Autodesk Inventor part; units mm, degrees
(part 3 of 4)
sketch "Sketch14" plane through (0, 0, 0) normal (0, 0, -1) x (-1, 0, 0)
  line L0 (-1.9956, 5.4384) -> (3.1347, 5.4384) construction
  line L1 (3.1347, 5.4384) -> (3.1347, -17.7526) construction
  line L2 (3.1347, -17.7526) -> (-1.9956, -17.7526) construction
  line L3 (-1.9956, -17.7526) -> (-1.9956, 5.4384) construction
  line L4 (4.75, -5.9162) -> (4.75, -5.8379)
  line L5 (4.75, -4.9221) -> (4.75, -4.8438)
  line L6 (5.6579, -4.9221) -> (5.6579, -5.8379)
  line L7 (4.75, -4.9221) -> (5.6579, -4.9221)
  line L8 (5.7362, -4.8438) -> (4.75, -4.8438)
  line L9 (5.7362, -5.9162) -> (5.7362, -4.8438)
  line L10 (5.6579, -5.8379) -> (4.75, -5.8379)
  line L11 (4.75, -5.9162) -> (5.7362, -5.9162)
  line L12 (4.55, -5.9162) -> (4.55, -5.8379)
  line L13 (4.55, -4.9221) -> (4.55, -4.8438)
  line L14 (4.55, -5.8379) -> (3.6421, -5.8379)
  line L15 (3.5638, -5.9162) -> (4.55, -5.9162)
  line L16 (3.6421, -4.9221) -> (4.55, -4.9221)
  line L17 (4.55, -4.8438) -> (3.5638, -4.8438)
  line L18 (3.6421, -5.8379) -> (3.6421, -4.9221)
  line L19 (3.5638, -4.8438) -> (3.5638, -5.9162)
  line L20 (4.55, -5.8379) -> (3.6421, -5.8379)
  line L21 (3.6421, -5.8379) -> (3.6421, -4.9221)
  line L22 (3.6421, -4.9221) -> (4.55, -4.9221)
  line L23 (4.55, -4.9221) -> (4.55, -4.8438)
  line L24 (4.55, -4.8438) -> (3.5638, -4.8438)
  line L25 (3.5638, -4.8438) -> (3.5638, -5.9162)
  line L26 (3.5638, -5.9162) -> (4.55, -5.9162)
  line L27 (4.55, -5.9162) -> (4.55, -5.8379)
  line L28 (4.75, -4.8438) -> (4.75, -4.9221)
  line L29 (4.75, -4.9221) -> (5.6579, -4.9221)
  line L30 (5.6579, -4.9221) -> (5.6579, -5.8379)
  line L31 (5.6579, -5.8379) -> (4.75, -5.8379)
  line L32 (4.75, -5.8379) -> (4.75, -5.9162)
  line L33 (4.75, -5.9162) -> (5.7362, -5.9162)
  line L34 (5.7362, -5.9162) -> (5.7362, -4.8438)
  line L35 (5.7362, -4.8438) -> (4.75, -4.8438)
  line L36 (-3.3239, 5.3849) -> (-3.3239, 5.4632)
  line L37 (-4.2318, 5.3849) -> (-3.3239, 5.3849)
  line L38 (-3.3239, 5.4632) -> (-4.3101, 5.4632)
  line L39 (-3.1239, 5.3849) -> (-3.1239, 5.4632)
  line L40 (-4.2318, 4.4692) -> (-4.2318, 5.3849)
  line L41 (-3.3239, 4.4692) -> (-4.2318, 4.4692)
  line L42 (-4.3101, 5.4632) -> (-4.3101, 4.3909)
  line L43 (-4.3101, 4.3909) -> (-3.3239, 4.3909)
  line L44 (-3.3239, 4.3909) -> (-3.3239, 4.4692)
  line L45 (-3.1239, 5.3849) -> (-2.2161, 5.3849)
  line L46 (-2.1378, 5.4632) -> (-3.1239, 5.4632)
  line L47 (-3.1239, 4.3909) -> (-3.1239, 4.4692)
  line L48 (-2.2161, 5.3849) -> (-2.2161, 4.4692)
  line L49 (-2.1378, 4.3909) -> (-2.1378, 5.4632)
  line L50 (-3.1239, 4.3909) -> (-2.1378, 4.3909)
  line L51 (-2.2161, 4.4692) -> (-3.1239, 4.4692)
  line L52 (-4.2318, 2.9331) -> (-4.2318, 3.8488)
  line L53 (-4.3101, 3.9271) -> (-4.3101, 2.8547)
  line L54 (-3.3239, 3.9271) -> (-4.3101, 3.9271)
  line L55 (-3.3239, 3.8488) -> (-3.3239, 3.9271)
  line L56 (-4.2318, 3.8488) -> (-3.3239, 3.8488)
  line L57 (-4.3101, 2.8547) -> (-3.3239, 2.8547)
  line L58 (-3.3239, 2.9331) -> (-4.2318, 2.9331)
  line L59 (-3.3239, 2.8547) -> (-3.3239, 2.9331)
  line L60 (-3.1239, 3.8488) -> (-3.1239, 3.9271)
  line L61 (-3.1239, 3.8488) -> (-2.2161, 3.8488)
  line L62 (-2.1378, 3.9271) -> (-3.1239, 3.9271)
  line L63 (-3.1239, 2.8547) -> (-3.1239, 2.9331)
  line L64 (-2.2161, 3.8488) -> (-2.2161, 2.9331)
  line L65 (-2.1378, 2.8547) -> (-2.1378, 3.9271)
  line L66 (-3.1239, 2.8547) -> (-2.1378, 2.8547)
  line L67 (-2.2161, 2.9331) -> (-3.1239, 2.9331)
  line L68 (-4.2318, 1.4571) -> (-4.2318, 2.3729)
  line L69 (-4.3101, 2.4512) -> (-4.3101, 1.3788)
  line L70 (-3.3239, 2.4512) -> (-4.3101, 2.4512)
  line L71 (-3.3239, 2.3729) -> (-3.3239, 2.4512)
  line L72 (-4.2318, 2.3729) -> (-3.3239, 2.3729)
  line L73 (-4.3101, 1.3788) -> (-3.3239, 1.3788)
  line L74 (-3.3239, 1.4571) -> (-4.2318, 1.4571)
  line L75 (-3.3239, 1.3788) -> (-3.3239, 1.4571)
  line L76 (-3.1239, 2.3729) -> (-3.1239, 2.4512)
  line L77 (-3.1239, 2.3729) -> (-2.2161, 2.3729)
  line L78 (-2.1378, 2.4512) -> (-3.1239, 2.4512)
  line L79 (-3.1239, 1.3788) -> (-3.1239, 1.4571)
  line L80 (-2.2161, 2.3729) -> (-2.2161, 1.4571)
  line L81 (-2.1378, 1.3788) -> (-2.1378, 2.4512)
  line L82 (-3.1239, 1.3788) -> (-2.1378, 1.3788)
  line L83 (-2.2161, 1.4571) -> (-3.1239, 1.4571)
  line L84 (-4.2318, -0.0188) -> (-4.2318, 0.8969)
  line L85 (-4.3101, 0.9753) -> (-4.3101, -0.0971)
  line L86 (-3.3239, 0.9753) -> (-4.3101, 0.9753)
  line L87 (-3.3239, 0.8969) -> (-3.3239, 0.9753)
  line L88 (-4.2318, 0.8969) -> (-3.3239, 0.8969)
  line L89 (-4.3101, -0.0971) -> (-3.3239, -0.0971)
  line L90 (-3.3239, -0.0188) -> (-4.2318, -0.0188)
  line L91 (-3.3239, -0.0971) -> (-3.3239, -0.0188)
  line L92 (-3.1239, 0.8969) -> (-3.1239, 0.9753)
  line L93 (-3.1239, 0.8969) -> (-2.2161, 0.8969)
  line L94 (-2.1378, 0.9753) -> (-3.1239, 0.9753)
  line L95 (-3.1239, -0.0971) -> (-3.1239, -0.0188)
  line L96 (-2.2161, 0.8969) -> (-2.2161, -0.0188)
  line L97 (-2.1378, -0.0971) -> (-2.1378, 0.9753)
  line L98 (-3.1239, -0.0971) -> (-2.1378, -0.0971)
  line L99 (-2.2161, -0.0188) -> (-3.1239, -0.0188)
  line L100 (-4.2318, -1.5262) -> (-4.2318, -0.6105)
  line L101 (-4.3101, -0.5322) -> (-4.3101, -1.6045)
  line L102 (-3.3239, -0.5322) -> (-4.3101, -0.5322)
  line L103 (-3.3239, -0.6105) -> (-3.3239, -0.5322)
  line L104 (-4.2318, -0.6105) -> (-3.3239, -0.6105)
  line L105 (-4.3101, -1.6045) -> (-3.3239, -1.6045)
  line L106 (-3.3239, -1.5262) -> (-4.2318, -1.5262)
  line L107 (-3.3239, -1.6045) -> (-3.3239, -1.5262)
  line L108 (-3.1239, -0.6105) -> (-3.1239, -0.5322)
  line L109 (-3.1239, -0.6105) -> (-2.2161, -0.6105)
  line L110 (-2.1378, -0.5322) -> (-3.1239, -0.5322)
  line L111 (-3.1239, -1.6045) -> (-3.1239, -1.5262)
  line L112 (-2.2161, -0.6105) -> (-2.2161, -1.5262)
  line L113 (-2.1378, -1.6045) -> (-2.1378, -0.5322)
  line L114 (-3.1239, -1.6045) -> (-2.1378, -1.6045)
  line L115 (-2.2161, -1.5262) -> (-3.1239, -1.5262)
  spline S0 degree 2 poles (-1.4607, 4.3962) (-1.686, 4.3962) (-1.9502, 4.6685) (-1.9502, 4.9149) knots 0 0 0 1 2 2 2
  spline S1 degree 2 poles (-1.9502, 4.9149) (-1.9502, 5.1523) (-1.6852, 5.4351) (-1.4599, 5.4351) knots 0 0 0 1 2 2 2
  spline S2 degree 2 poles (-1.4599, 5.4351) (-1.4007, 5.4351) (-1.3051, 5.4214) (-1.2614, 5.41) knots 0 0 0 1 2 2 2
  spline S3 degree 2 poles (-1.2614, 5.41) (-1.2273, 5.3995) (-1.1471, 5.3646) (-1.122, 5.3517) knots 0 0 0 1 2 2 2
  line L116 (-1.122, 5.3517) -> (-1.122, 5.1134)
  line L117 (-1.122, 5.1134) -> (-1.1471, 5.1134)
  spline S4 degree 2 poles (-1.1471, 5.1134) (-1.1657, 5.1296) (-1.2208, 5.175) (-1.2557, 5.1961) knots 0 0 0 1 2 2 2
  spline S5 degree 2 poles (-1.2557, 5.1961) (-1.2905, 5.218) (-1.374, 5.2479) (-1.4202, 5.2479) knots 0 0 0 1 2 2 2
  spline S6 degree 2 poles (-1.4202, 5.2479) (-1.4745, 5.2479) (-1.5644, 5.2139) (-1.6058, 5.171) knots 0 0 0 1 2 2 2
  spline S7 degree 2 poles (-1.6058, 5.171) (-1.643, 5.1329) (-1.6909, 5.0024) (-1.6909, 4.9141) knots 0 0 0 1 2 2 2
  spline S8 degree 2 poles (-1.6909, 4.9141) (-1.6909, 4.8209) (-1.6414, 4.6936) (-1.6009, 4.6547) knots 0 0 0 1 2 2 2
  spline S9 degree 2 poles (-1.6009, 4.6547) (-1.562, 4.6167) (-1.4664, 4.5834) (-1.4186, 4.5834) knots 0 0 0 1 2 2 2
  spline S10 degree 2 poles (-1.4186, 4.5834) (-1.3691, 4.5834) (-1.2792, 4.6167) (-1.2484, 4.6369) knots 0 0 0 1 2 2 2
  spline S11 degree 2 poles (-1.2484, 4.6369) (-1.2144, 4.6572) (-1.1633, 4.7001) (-1.1447, 4.7171) knots 0 0 0 1 2 2 2
  line L118 (-1.1447, 4.7171) -> (-1.122, 4.7171)
  line L119 (-1.122, 4.7171) -> (-1.122, 4.4821)
  spline S12 degree 2 poles (-1.122, 4.4821) (-1.1495, 4.4692) (-1.2216, 4.4368) (-1.2605, 4.4254) knots 0 0 0 1 2 2 2
  spline S13 degree 2 poles (-1.2605, 4.4254) (-1.3075, 4.4108) (-1.3894, 4.3962) (-1.4607, 4.3962) knots 0 0 0 1 2 2 2
  spline S14 degree 2 poles (-0.2435, 4.6936) (-0.2435, 4.6296) (-0.297, 4.5186) (-0.3481, 4.4781) knots 0 0 0 1 2 2 2
  spline S15 degree 2 poles (-0.3481, 4.4781) (-0.3991, 4.4376) (-0.5458, 4.3922) (-0.6406, 4.3922) knots 0 0 0 1 2 2 2
  spline S16 degree 2 poles (-0.6406, 4.3922) (-0.7419, 4.3922) (-0.8934, 4.4384) (-0.9421, 4.4781) knots 0 0 0 1 2 2 2
  spline S17 degree 2 poles (-0.9421, 4.4781) (-0.9899, 4.5178) (-1.0353, 4.6256) (-1.0353, 4.6855) knots 0 0 0 1 2 2 2
  spline S18 degree 2 poles (-1.0353, 4.6855) (-1.0353, 4.7714) (-0.9404, 4.8857) (-0.8505, 4.9238) knots 0 0 0 1 2 2 2
  line L120 (-0.8505, 4.9238) -> (-0.8505, 4.9278)
  spline S19 degree 2 poles (-0.8505, 4.9278) (-0.9388, 4.9708) (-1.0085, 5.0932) (-1.0085, 5.1685) knots 0 0 0 1 2 2 2
  spline S20 degree 2 poles (-1.0085, 5.1685) (-1.0085, 5.2236) (-0.9599, 5.3201) (-0.9121, 5.3581) knots 0 0 0 1 2 2 2
  spline S21 degree 2 poles (-0.9121, 5.3581) (-0.8659, 5.3946) (-0.7257, 5.4384) (-0.6382, 5.4384) knots 0 0 0 1 2 2 2
  spline S22 degree 2 poles (-0.6382, 5.4384) (-0.5458, 5.4384) (-0.408, 5.3987) (-0.3635, 5.3663) knots 0 0 0 1 2 2 2
  spline S23 degree 2 poles (-0.3635, 5.3663) (-0.3181, 5.3338) (-0.2695, 5.2398) (-0.2695, 5.1855) knots 0 0 0 1 2 2 2
  spline S24 degree 2 poles (-0.2695, 5.1855) (-0.2695, 5.1142) (-0.3521, 5) (-0.4372, 4.9603) knots 0 0 0 1 2 2 2
  line L121 (-0.4372, 4.9603) -> (-0.4372, 4.957)
  spline S25 degree 2 poles (-0.4372, 4.957) (-0.3375, 4.9165) (-0.2435, 4.7852) (-0.2435, 4.6936) knots 0 0 0 1 2 2 2
  spline S26 degree 2 poles (-0.4915, 4.6831) (-0.4915, 4.7325) (-0.5336, 4.7844) (-0.6017, 4.8176) knots 0 0 0 1 2 2 2
  spline S27 degree 2 poles (-0.6017, 4.8176) (-0.6212, 4.8265) (-0.6949, 4.8549) (-0.7233, 4.8671) knots 0 0 0 1 2 2 2
  spline S28 degree 2 poles (-0.7233, 4.8671) (-0.7492, 4.8411) (-0.7905, 4.7633) (-0.7905, 4.7171) knots 0 0 0 1 2 2 2
  spline S29 degree 2 poles (-0.7905, 4.7171) (-0.7905, 4.6475) (-0.7014, 4.564) (-0.6293, 4.564) knots 0 0 0 1 2 2 2
  spline S30 degree 2 poles (-0.6293, 4.564) (-0.609, 4.564) (-0.5588, 4.5769) (-0.5393, 4.5899) knots 0 0 0 1 2 2 2
  spline S31 degree 2 poles (-0.5393, 4.5899) (-0.5174, 4.6053) (-0.4915, 4.6475) (-0.4915, 4.6831) knots 0 0 0 1 2 2 2
  spline S32 degree 2 poles (-0.5134, 5.1564) (-0.5134, 5.2074) (-0.5806, 5.2682) (-0.6382, 5.2682) knots 0 0 0 1 2 2 2
  spline S33 degree 2 poles (-0.6382, 5.2682) (-0.6933, 5.2682) (-0.7605, 5.2131) (-0.7605, 5.1726) knots 0 0 0 1 2 2 2
  spline S34 degree 2 poles (-0.7605, 5.1726) (-0.7605, 5.1329) (-0.72, 5.0834) (-0.6771, 5.0632) knots 0 0 0 1 2 2 2
  spline S35 degree 2 poles (-0.6771, 5.0632) (-0.6584, 5.0534) (-0.6066, 5.0332) (-0.5636, 5.017) knots 0 0 0 1 2 2 2
  spline S36 degree 2 poles (-0.5636, 5.017) (-0.5377, 5.051) (-0.5134, 5.115) (-0.5134, 5.1564) knots 0 0 0 1 2 2 2
  spline S37 degree 2 poles (-0.9996, 3.4149) (-0.9996, 3.2747) (-1.122, 3.0543) (-1.2152, 2.9951) knots 0 0 0 1 2 2 2
  spline S38 degree 2 poles (-1.2152, 2.9951) (-1.293, 2.9449) (-1.4761, 2.9157) (-1.579, 2.9157) knots 0 0 0 1 2 2 2
  line L122 (-1.579, 2.9157) -> (-1.8918, 2.9157)
  line L123 (-1.8918, 2.9157) -> (-1.8918, 3.9157)
  line L124 (-1.8918, 3.9157) -> (-1.5823, 3.9157)
  spline S39 degree 2 poles (-1.5823, 3.9157) (-1.4769, 3.9157) (-1.293, 3.8889) (-1.2119, 3.8371) knots 0 0 0 1 2 2 2
  spline S40 degree 2 poles (-1.2119, 3.8371) (-1.1139, 3.7739) (-0.9996, 3.5599) (-0.9996, 3.4149) knots 0 0 0 1 2 2 2
  spline S41 degree 2 poles (-1.2573, 3.4165) (-1.2573, 3.5154) (-1.3254, 3.6564) (-1.3951, 3.6961) knots 0 0 0 1 2 2 2
  spline S42 degree 2 poles (-1.3951, 3.6961) (-1.4461, 3.7236) (-1.5579, 3.7293) (-1.6357, 3.7293) knots 0 0 0 1 2 2 2
  line L125 (-1.6357, 3.7293) -> (-1.6406, 3.7293)
  line L126 (-1.6406, 3.7293) -> (-1.6406, 3.1029)
  line L127 (-1.6406, 3.1029) -> (-1.6357, 3.1029)
  spline S43 degree 2 poles (-1.6357, 3.1029) (-1.5515, 3.1029) (-1.4356, 3.1086) (-1.3829, 3.1418) knots 0 0 0 1 2 2 2
  spline S44 degree 2 poles (-1.3829, 3.1418) (-1.3213, 3.1807) (-1.2573, 3.3176) (-1.2573, 3.4165) knots 0 0 0 1 2 2 2
  line L128 (-0.1625, 2.9157) -> (-0.8229, 2.9157)
  line L129 (-0.8229, 2.9157) -> (-0.8229, 3.0899)
  line L130 (-0.8229, 3.0899) -> (-0.6122, 3.0899)
  line L131 (-0.6122, 3.0899) -> (-0.6122, 3.6191)
  line L132 (-0.6122, 3.6191) -> (-0.8229, 3.6191)
  line L133 (-0.8229, 3.6191) -> (-0.8229, 3.782)
  spline S45 degree 2 poles (-0.8229, 3.782) (-0.7767, 3.782) (-0.6852, 3.7941) (-0.6576, 3.8071) knots 0 0 0 1 2 2 2
  spline S46 degree 2 poles (-0.6576, 3.8071) (-0.626, 3.8233) (-0.5904, 3.8776) (-0.5871, 3.9181) knots 0 0 0 1 2 2 2
  line L134 (-0.5871, 3.9181) -> (-0.3683, 3.9181)
  line L135 (-0.3683, 3.9181) -> (-0.3683, 3.0899)
  line L136 (-0.3683, 3.0899) -> (-0.1625, 3.0899)
  line L137 (-0.1625, 3.0899) -> (-0.1625, 2.9157)
  line L138 (-0.968, 1.4157) -> (-1.2735, 1.4157)
  line L139 (-1.2735, 1.4157) -> (-1.5515, 1.7828)
  line L140 (-1.5515, 1.7828) -> (-1.6422, 1.7828)
  line L141 (-1.6422, 1.7828) -> (-1.6422, 1.4157)
  line L142 (-1.6422, 1.4157) -> (-1.8918, 1.4157)
  line L143 (-1.8918, 1.4157) -> (-1.8918, 2.4157)
  line L144 (-1.8918, 2.4157) -> (-1.4899, 2.4157)
  spline S47 degree 2 poles (-1.4899, 2.4157) (-1.4064, 2.4157) (-1.2832, 2.3946) (-1.2306, 2.3622) knots 0 0 0 1 2 2 2
  spline S48 degree 2 poles (-1.2306, 2.3622) (-1.1771, 2.3282) (-1.1139, 2.222) (-1.1139, 2.141) knots 0 0 0 1 2 2 2
  spline S49 degree 2 poles (-1.1139, 2.141) (-1.1139, 2.0267) (-1.2176, 1.8833) (-1.3043, 1.8411) knots 0 0 0 1 2 2 2
  line L145 (-1.3043, 1.8411) -> (-0.968, 1.4157)
  spline S50 degree 2 poles (-1.3716, 2.1094) (-1.3716, 2.1475) (-1.4007, 2.2017) (-1.434, 2.2163) knots 0 0 0 1 2 2 2
  spline S51 degree 2 poles (-1.434, 2.2163) (-1.4575, 2.2261) (-1.515, 2.2317) (-1.5579, 2.2317) knots 0 0 0 1 2 2 2
  line L146 (-1.5579, 2.2317) -> (-1.6422, 2.2317)
  line L147 (-1.6422, 2.2317) -> (-1.6422, 1.9627)
  line L148 (-1.6422, 1.9627) -> (-1.5701, 1.9627)
  spline S52 degree 2 poles (-1.5701, 1.9627) (-1.5182, 1.9627) (-1.4445, 1.9757) (-1.4194, 1.9959) knots 0 0 0 1 2 2 2
  spline S53 degree 2 poles (-1.4194, 1.9959) (-1.3951, 2.0154) (-1.3716, 2.0672) (-1.3716, 2.1094) knots 0 0 0 1 2 2 2
  line L149 (-0.1609, 1.4157) -> (-0.8959, 1.4157)
  line L150 (-0.8959, 1.4157) -> (-0.8959, 1.5786)
  spline S54 degree 2 poles (-0.8959, 1.5786) (-0.8027, 1.6531) (-0.6536, 1.7844) (-0.5977, 1.8436) knots 0 0 0 1 2 2 2
  spline S55 degree 2 poles (-0.5977, 1.8436) (-0.5239, 1.9205) (-0.4583, 2.0381) (-0.4583, 2.0996) knots 0 0 0 1 2 2 2
  spline S56 degree 2 poles (-0.4583, 2.0996) (-0.4583, 2.1693) (-0.5417, 2.2439) (-0.6163, 2.2439) knots 0 0 0 1 2 2 2
  spline S57 degree 2 poles (-0.6163, 2.2439) (-0.6544, 2.2439) (-0.7225, 2.2252) (-0.7573, 2.2107) knots 0 0 0 1 2 2 2
  spline S58 degree 2 poles (-0.7573, 2.2107) (-0.7913, 2.1953) (-0.84, 2.1628) (-0.8521, 2.1547) knots 0 0 0 1 2 2 2
  line L151 (-0.8521, 2.1547) -> (-0.8716, 2.1547)
  line L152 (-0.8716, 2.1547) -> (-0.8716, 2.3727)
  spline S59 degree 2 poles (-0.8716, 2.3727) (-0.8294, 2.393) (-0.6495, 2.4351) (-0.5661, 2.4351) knots 0 0 0 1 2 2 2
  spline S60 degree 2 poles (-0.5661, 2.4351) (-0.3878, 2.4351) (-0.2046, 2.2763) (-0.2046, 2.1329) knots 0 0 0 1 2 2 2
  spline S61 degree 2 poles (-0.2046, 2.1329) (-0.2046, 2.0445) (-0.2881, 1.8744) (-0.3845, 1.7771) knots 0 0 0 1 2 2 2
  spline S62 degree 2 poles (-0.3845, 1.7771) (-0.4453, 1.7171) (-0.5596, 1.6239) (-0.5847, 1.6045) knots 0 0 0 1 2 2 2
  line L153 (-0.5847, 1.6045) -> (-0.1609, 1.6045)
  line L154 (-0.1609, 1.6045) -> (-0.1609, 1.4157)
  line L155 (-0.968, -0.0843) -> (-1.2735, -0.0843)
  line L156 (-1.2735, -0.0843) -> (-1.5515, 0.2828)
  line L157 (-1.5515, 0.2828) -> (-1.6422, 0.2828)
  line L158 (-1.6422, 0.2828) -> (-1.6422, -0.0843)
  line L159 (-1.6422, -0.0843) -> (-1.8918, -0.0843)
  line L160 (-1.8918, -0.0843) -> (-1.8918, 0.9157)
  line L161 (-1.8918, 0.9157) -> (-1.4899, 0.9157)
  spline S63 degree 2 poles (-1.4899, 0.9157) (-1.4064, 0.9157) (-1.2832, 0.8946) (-1.2306, 0.8622) knots 0 0 0 1 2 2 2
  spline S64 degree 2 poles (-1.2306, 0.8622) (-1.1771, 0.8282) (-1.1139, 0.722) (-1.1139, 0.641) knots 0 0 0 1 2 2 2
  spline S65 degree 2 poles (-1.1139, 0.641) (-1.1139, 0.5267) (-1.2176, 0.3833) (-1.3043, 0.3411) knots 0 0 0 1 2 2 2
  line L162 (-1.3043, 0.3411) -> (-0.968, -0.0843)
  spline S66 degree 2 poles (-1.3716, 0.6094) (-1.3716, 0.6475) (-1.4007, 0.7017) (-1.434, 0.7163) knots 0 0 0 1 2 2 2
  spline S67 degree 2 poles (-1.434, 0.7163) (-1.4575, 0.7261) (-1.515, 0.7317) (-1.5579, 0.7317) knots 0 0 0 1 2 2 2
  line L163 (-1.5579, 0.7317) -> (-1.6422, 0.7317)
  line L164 (-1.6422, 0.7317) -> (-1.6422, 0.4627)
  line L165 (-1.6422, 0.4627) -> (-1.5701, 0.4627)
  spline S68 degree 2 poles (-1.5701, 0.4627) (-1.5182, 0.4627) (-1.4445, 0.4757) (-1.4194, 0.4959) knots 0 0 0 1 2 2 2
  spline S69 degree 2 poles (-1.4194, 0.4959) (-1.3951, 0.5154) (-1.3716, 0.5672) (-1.3716, 0.6094) knots 0 0 0 1 2 2 2
  spline S70 degree 2 poles (-0.186, 0.2188) (-0.186, 0.145) (-0.2403, 0.0243) (-0.293, -0.0179) knots 0 0 0 1 2 2 2
  spline S71 degree 2 poles (-0.293, -0.0179) (-0.3456, -0.06) (-0.4891, -0.1054) (-0.592, -0.1054) knots 0 0 0 1 2 2 2
  spline S72 degree 2 poles (-0.592, -0.1054) (-0.7087, -0.1054) (-0.8756, -0.0665) (-0.9283, -0.0422) knots 0 0 0 1 2 2 2
  line L166 (-0.9283, -0.0422) -> (-0.9283, 0.175)
  line L167 (-0.9283, 0.175) -> (-0.904, 0.175)
  spline S73 degree 2 poles (-0.904, 0.175) (-0.8489, 0.1402) (-0.7006, 0.0883) (-0.639, 0.0883) knots 0 0 0 1 2 2 2
  spline S74 degree 2 poles (-0.639, 0.0883) (-0.6025, 0.0883) (-0.5174, 0.1013) (-0.4883, 0.1223) knots 0 0 0 1 2 2 2
  spline S75 degree 2 poles (-0.4883, 0.1223) (-0.4656, 0.1393) (-0.438, 0.1888) (-0.438, 0.2333) knots 0 0 0 1 2 2 2
  spline S76 degree 2 poles (-0.438, 0.2333) (-0.438, 0.2779) (-0.4769, 0.3257) (-0.5093, 0.3371) knots 0 0 0 1 2 2 2
  spline S77 degree 2 poles (-0.5093, 0.3371) (-0.5417, 0.3484) (-0.6317, 0.3509) (-0.6665, 0.3509) knots 0 0 0 1 2 2 2
  line L168 (-0.6665, 0.3509) -> (-0.7095, 0.3509)
  line L169 (-0.7095, 0.3509) -> (-0.7095, 0.5267)
  line L170 (-0.7095, 0.5267) -> (-0.6698, 0.5267)
  spline S78 degree 2 poles (-0.6698, 0.5267) (-0.6244, 0.5267) (-0.5474, 0.5348) (-0.5207, 0.547) knots 0 0 0 1 2 2 2
  spline S79 degree 2 poles (-0.5207, 0.547) (-0.4939, 0.5599) (-0.4639, 0.6053) (-0.4639, 0.6442) knots 0 0 0 1 2 2 2
  spline S80 degree 2 poles (-0.4639, 0.6442) (-0.4639, 0.675) (-0.4923, 0.7131) (-0.5126, 0.7236) knots 0 0 0 1 2 2 2
  spline S81 degree 2 poles (-0.5126, 0.7236) (-0.5369, 0.7358) (-0.6017, 0.7439) (-0.6244, 0.7439) knots 0 0 0 1 2 2 2
  spline S82 degree 2 poles (-0.6244, 0.7439) (-0.6609, 0.7439) (-0.7379, 0.7269) (-0.7735, 0.7131) knots 0 0 0 1 2 2 2
  spline S83 degree 2 poles (-0.7735, 0.7131) (-0.8019, 0.7026) (-0.8635, 0.6685) (-0.878, 0.6596) knots 0 0 0 1 2 2 2
  line L171 (-0.878, 0.6596) -> (-0.8991, 0.6596)
  line L172 (-0.8991, 0.6596) -> (-0.8991, 0.8735)
  spline S84 degree 2 poles (-0.8991, 0.8735) (-0.8473, 0.8954) (-0.6722, 0.9368) (-0.5806, 0.9368) knots 0 0 0 1 2 2 2
  spline S85 degree 2 poles (-0.5806, 0.9368) (-0.4915, 0.9368) (-0.3602, 0.906) (-0.314, 0.876) knots 0 0 0 1 2 2 2
  spline S86 degree 2 poles (-0.314, 0.876) (-0.263, 0.8444) (-0.2119, 0.7471) (-0.2119, 0.6863) knots 0 0 0 1 2 2 2
  spline S87 degree 2 poles (-0.2119, 0.6863) (-0.2119, 0.6004) (-0.3108, 0.4724) (-0.3918, 0.4538) knots 0 0 0 1 2 2 2
  line L173 (-0.3918, 0.4538) -> (-0.3918, 0.444)
  spline S88 degree 2 poles (-0.3918, 0.444) (-0.3562, 0.4392) (-0.2881, 0.4133) (-0.2557, 0.3841) knots 0 0 0 1 2 2 2
  spline S89 degree 2 poles (-0.2557, 0.3841) (-0.2257, 0.3581) (-0.186, 0.2755) (-0.186, 0.2188) knots 0 0 0 1 2 2 2
  line L174 (-0.968, -1.5843) -> (-1.2735, -1.5843)
  line L175 (-1.2735, -1.5843) -> (-1.5515, -1.2172)
  line L176 (-1.5515, -1.2172) -> (-1.6422, -1.2172)
  line L177 (-1.6422, -1.2172) -> (-1.6422, -1.5843)
  line L178 (-1.6422, -1.5843) -> (-1.8918, -1.5843)
  line L179 (-1.8918, -1.5843) -> (-1.8918, -0.5843)
  line L180 (-1.8918, -0.5843) -> (-1.4899, -0.5843)
  spline S90 degree 2 poles (-1.4899, -0.5843) (-1.4064, -0.5843) (-1.2832, -0.6054) (-1.2306, -0.6378) knots 0 0 0 1 2 2 2
  spline S91 degree 2 poles (-1.2306, -0.6378) (-1.1771, -0.6718) (-1.1139, -0.778) (-1.1139, -0.859) knots 0 0 0 1 2 2 2
  spline S92 degree 2 poles (-1.1139, -0.859) (-1.1139, -0.9733) (-1.2176, -1.1167) (-1.3043, -1.1589) knots 0 0 0 1 2 2 2
  line L181 (-1.3043, -1.1589) -> (-0.968, -1.5843)
  spline S93 degree 2 poles (-1.3716, -0.8906) (-1.3716, -0.8525) (-1.4007, -0.7983) (-1.434, -0.7837) knots 0 0 0 1 2 2 2
  spline S94 degree 2 poles (-1.434, -0.7837) (-1.4575, -0.7739) (-1.515, -0.7683) (-1.5579, -0.7683) knots 0 0 0 1 2 2 2
  line L182 (-1.5579, -0.7683) -> (-1.6422, -0.7683)
  line L183 (-1.6422, -0.7683) -> (-1.6422, -1.0373)
  line L184 (-1.6422, -1.0373) -> (-1.5701, -1.0373)
  spline S95 degree 2 poles (-1.5701, -1.0373) (-1.5182, -1.0373) (-1.4445, -1.0243) (-1.4194, -1.0041) knots 0 0 0 1 2 2 2
  spline S96 degree 2 poles (-1.4194, -1.0041) (-1.3951, -0.9846) (-1.3716, -0.9328) (-1.3716, -0.8906) knots 0 0 0 1 2 2 2
  line L185 (-0.1487, -1.3509) -> (-0.284, -1.3509)
  line L186 (-0.284, -1.3509) -> (-0.284, -1.5867)
  line L187 (-0.284, -1.5867) -> (-0.5263, -1.5867)
  line L188 (-0.5263, -1.5867) -> (-0.5263, -1.3509)
  line L189 (-0.5263, -1.3509) -> (-0.9672, -1.3509)
  line L190 (-0.9672, -1.3509) -> (-0.9672, -1.1645)
  line L191 (-0.9672, -1.1645) -> (-0.5344, -0.5843)
  line L192 (-0.5344, -0.5843) -> (-0.284, -0.5843)
  line L193 (-0.284, -0.5843) -> (-0.284, -1.171)
  line L194 (-0.284, -1.171) -> (-0.1487, -1.171)
  line L195 (-0.1487, -1.171) -> (-0.1487, -1.3509)
  line L196 (-0.5263, -1.171) -> (-0.5263, -0.8307)
  line L197 (-0.5263, -0.8307) -> (-0.78, -1.171)
  line L198 (-0.78, -1.171) -> (-0.5263, -1.171)
  point P0 (0, 0)
  point P1 (5.6, -4.98)
  point P2 (-2.2739, 5.3271)
  point P3 (-2.2739, 3.7909)
  point P4 (-2.2739, 2.315)
  point P5 (-2.2739, 0.8391)
  point P6 (-2.2739, -0.6684)
  constraints: 192 end point, 2 other
extrude "Extrusion14" add sketch "Sketch14" along normal blind 0.1 separate body contours L37 L40 L41 L44 L43 L42 L38 L36 | L39 L46 L49 L50 L47 L51 L48 L45 | L58 L59 L57 L53 L54 L55 L56 L52 | L60 L62 L65 L66 L63 L67 L64 L61 | L74 L75 L73 L69 L70 L71 L72 L68 | L76 L78 L81 L82 L79 L83 L80 L77 | L90 L91 L89 L85 L86 L87 L88 L84 | L92 L94 L97 L98 L95 L99 L96 L93 | L106 L107 L105 L101 L102 L103 L104 L100 | L108 L110 L113 L114 L111 L115 L112 L109 | S0 S1 S2 S3 L116 L117 S4 S5 S6 S7 S8 S9 S10 S11 L118 L119 S12 S13 | S14 S15 S16 S17 S18 L120 S19 S20 S21 S22 S23 S24 L121 S25 | S37 S38 L122 L123 L124 S39 S40 | L128 L129 L130 L131 L132 L133 S45 S46 L134 L135 L136 L137 | L138 L139 L140 L141 L142 L143 L144 S47 S48 S49 L145 | L149 L150 S54 S55 S56 S57 S58 L151 L152 S59 S60 S61 S62 L153 L154 | L155 L156 L157 L158 L159 L160 L161 S63 S64 S65 L162 | S70 S71 S72 L166 L167 S73 S74 S75 S76 S77 L168 L169 L170 S78 S79 S80 S81 S82 S83 L171 L172 S84 S85 S86 S87 L173 S88 S89 | L174 L175 L176 L177 L178 L179 L180 S90 S91 S92 L181 | L185 L186 L187 L188 L189 L190 L191 L192 L193 L194 L195
sketch "Sketch15" plane through (0, 0, 0) normal (0, 0, -1) x (-1, 0, 0)
  line L0 (3.7, 1.72) -> (3.7, 0.92)
  line L1 (5.6, 1.72) -> (3.7, 1.72)
  line L2 (3.7, 0.92) -> (5.6, 0.92)
  line L3 (5.6, 0.92) -> (5.6, 1.72)
  line L4 (-4.2318, 5.3849) -> (-3.3239, 5.3849)
  line L5 (-4.2318, 5.3849) -> (-2.2161, 5.3849)
  line L6 (-2.2161, 4.4692) -> (-3.1239, 4.4692)
  line L7 (-2.2161, 5.3849) -> (-2.2161, 4.4692)
  line L8 (-4.2318, 4.4692) -> (-4.2318, 5.3849)
  line L9 (-2.2161, 4.4692) -> (-4.2318, 4.4692)
  line L10 (-4.2318, 4.4692) -> (-4.2318, 5.3849)
  line L11 (-2.2907, 5.3103) -> (-4.1571, 5.3103)
  line L12 (-4.1571, 5.3103) -> (-4.1571, 4.5439)
  line L13 (-4.1571, 4.5439) -> (-2.2907, 4.5439)
  line L14 (-2.2907, 4.5439) -> (-2.2907, 5.3103)
  line L15 (-2.2907, 3.7924) -> (-4.1571, 3.7924)
  line L16 (-4.1571, 3.7924) -> (-4.1571, 3.026)
  line L17 (-4.1571, 3.026) -> (-2.2907, 3.026)
  line L18 (-2.2907, 3.026) -> (-2.2907, 3.7924)
  line L19 (-2.2907, 2.3165) -> (-4.1571, 2.3165)
  line L20 (-4.1571, 2.3165) -> (-4.1571, 1.5501)
  line L21 (-4.1571, 1.5501) -> (-2.2907, 1.5501)
  line L22 (-2.2907, 1.5501) -> (-2.2907, 2.3165)
  line L23 (-2.2907, 0.8182) -> (-4.1571, 0.8182)
  line L24 (-4.1571, 0.8182) -> (-4.1571, 0.0518)
  line L25 (-4.1571, 0.0518) -> (-2.2907, 0.0518)
  line L26 (-2.2907, 0.0518) -> (-2.2907, 0.8182)
  line L27 (-2.2907, -0.6669) -> (-4.1571, -0.6669)
  line L28 (-4.1571, -0.6669) -> (-4.1571, -1.4333)
  line L29 (-4.1571, -1.4333) -> (-2.2907, -1.4333)
  line L30 (-2.2907, -1.4333) -> (-2.2907, -0.6669)
  point P0 (0, 0)
  point P1 (-2.2161, 2.9331)
  point P2 (-2.2161, 1.4571)
  point P3 (-2.2161, -0.0188)
  point P4 (-2.2161, -1.5262)
  constraints: 48 end point, 18 perpendicular, 1 horizontal, 3 other
extrude "Extrusion15" add sketch "Sketch15" along normal up to surface (1 mm away) separate body contours L14 L13 L12 L11 | L18 L17 L16 L15 | L22 L21 L20 L19 | L26 L25 L24 L23 | L30 L29 L28 L27
chamfer "Chamfer4" distance 0.1 angle 45 20 edges at (4.1571, 1.9333, -1) (3.2239, 1.5501, -1) (2.2907, 1.9333, -1) (3.2239, 2.3165, -1) (4.1571, 0.435, -1) (3.2239, 0.0518, -1) (2.2907, 0.435, -1) (3.2239, 0.8182, -1) (4.1571, -1.0501, -1) (3.2239, -0.6669, -1) (3.2239, -1.4333, -1) (2.2907, -1.0501, -1) (4.1571, 3.4092, -1) (3.2239, 3.026, -1) (2.2907, 3.4092, -1) (3.2239, 3.7924, -1) (3.2239, 4.5439, -1) (2.2907, 4.9271, -1) (3.2239, 5.3103, -1) (4.1571, 4.9271, -1)
sketch "Sketch16" plane through (0, 0, 0) normal (0, 0, -1) x (-1, 0, 0)
  line L0 (-14.6361, -2.8124) -> (1.3623, -2.8124) construction
  line L1 (1.3623, -2.8124) -> (1.3623, -4.8966) construction
  line L2 (1.3623, -4.8966) -> (-14.6361, -4.8966) construction
  line L3 (-14.6361, -4.8966) -> (-14.6361, -2.8124) construction
  spline S0 degree 2 poles (-12.9894, -3.8545) (-12.9894, -4.1138) (-13.0721, -4.5028) (-13.1645, -4.6341) knots 0 0 0 1 2 2 2
  spline S1 degree 2 poles (-13.1645, -4.6341) (-13.2552, -4.7637) (-13.5486, -4.8966) (-13.7593, -4.8966) knots 0 0 0 1 2 2 2
  spline S2 degree 2 poles (-13.7593, -4.8966) (-13.9716, -4.8966) (-14.2633, -4.7637) (-14.3557, -4.6308) knots 0 0 0 1 2 2 2
  spline S3 degree 2 poles (-14.3557, -4.6308) (-14.4481, -4.4996) (-14.5307, -4.1138) (-14.5307, -3.8545) knots 0 0 0 1 2 2 2
  spline S4 degree 2 poles (-14.5307, -3.8545) (-14.5307, -3.5887) (-14.4481, -3.2127) (-14.3541, -3.0765) knots 0 0 0 1 2 2 2
  spline S5 degree 2 poles (-14.3541, -3.0765) (-14.2601, -2.9436) (-13.9635, -2.814) (-13.7593, -2.814) knots 0 0 0 1 2 2 2
  spline S6 degree 2 poles (-13.7593, -2.814) (-13.5437, -2.814) (-13.2552, -2.9501) (-13.1628, -3.0846) knots 0 0 0 1 2 2 2
  spline S7 degree 2 poles (-13.1628, -3.0846) (-13.0721, -3.2159) (-12.9894, -3.6033) (-12.9894, -3.8545) knots 0 0 0 1 2 2 2
  spline S8 degree 2 poles (-13.4935, -3.8545) (-13.4935, -3.4834) (-13.615, -3.1835) (-13.7593, -3.1835) knots 0 0 0 1 2 2 2
  spline S9 degree 2 poles (-13.7593, -3.1835) (-13.9035, -3.1835) (-14.0267, -3.4834) (-14.0267, -3.8561) knots 0 0 0 1 2 2 2
  spline S10 degree 2 poles (-14.0267, -3.8561) (-14.0267, -4.2224) (-13.9035, -4.5271) (-13.7593, -4.5271) knots 0 0 0 1 2 2 2
  spline S11 degree 2 poles (-13.7593, -4.5271) (-13.6166, -4.5271) (-13.4935, -4.2224) (-13.4935, -3.8545) knots 0 0 0 1 2 2 2
  line L4 (-12.2179, -4.8545) -> (-12.6928, -4.8545)
  line L5 (-12.6928, -4.8545) -> (-12.6928, -4.3261)
  line L6 (-12.6928, -4.3261) -> (-12.2179, -4.3261)
  line L7 (-12.2179, -4.3261) -> (-12.2179, -4.8545)
  spline S12 degree 2 poles (-10.4043, -3.7427) (-10.4043, -3.9971) (-10.5226, -4.4218) (-10.6474, -4.5741) knots 0 0 0 1 2 2 2
  spline S13 degree 2 poles (-10.6474, -4.5741) (-10.7771, -4.7281) (-11.1596, -4.8934) (-11.4384, -4.8934) knots 0 0 0 1 2 2 2
  spline S14 degree 2 poles (-11.4384, -4.8934) (-11.5324, -4.8934) (-11.7366, -4.8691) (-11.7706, -4.8594) knots 0 0 0 1 2 2 2
  line L8 (-11.7706, -4.8594) -> (-11.7706, -4.4671)
  line L9 (-11.7706, -4.4671) -> (-11.7317, -4.4671)
  spline S15 degree 2 poles (-11.7317, -4.4671) (-11.6944, -4.4866) (-11.5551, -4.5287) (-11.4335, -4.5287) knots 0 0 0 1 2 2 2
  spline S16 degree 2 poles (-11.4335, -4.5287) (-11.3346, -4.5287) (-11.1515, -4.4769) (-11.0867, -4.4201) knots 0 0 0 1 2 2 2
  spline S17 degree 2 poles (-11.0867, -4.4201) (-11.017, -4.3602) (-10.9262, -4.1835) (-10.91, -4.0506) knots 0 0 0 1 2 2 2
  spline S18 degree 2 poles (-10.91, -4.0506) (-11.017, -4.1171) (-11.2017, -4.1884) (-11.3395, -4.1884) knots 0 0 0 1 2 2 2
  spline S19 degree 2 poles (-11.3395, -4.1884) (-11.4416, -4.1884) (-11.6312, -4.1333) (-11.709, -4.0749) knots 0 0 0 1 2 2 2
  spline S20 degree 2 poles (-11.709, -4.0749) (-11.8128, -3.9955) (-11.9343, -3.7411) (-11.9343, -3.5401) knots 0 0 0 1 2 2 2
  spline S21 degree 2 poles (-11.9343, -3.5401) (-11.9343, -3.3829) (-11.8273, -3.1187) (-11.7301, -3.0214) knots 0 0 0 1 2 2 2
  spline S22 degree 2 poles (-11.7301, -3.0214) (-11.6329, -2.9242) (-11.3508, -2.814) (-11.1774, -2.814) knots 0 0 0 1 2 2 2
  spline S23 degree 2 poles (-11.1774, -2.814) (-11.0024, -2.814) (-10.7317, -2.9112) (-10.6345, -3.0133) knots 0 0 0 1 2 2 2
  spline S24 degree 2 poles (-10.6345, -3.0133) (-10.521, -3.1268) (-10.4043, -3.4866) (-10.4043, -3.7427) knots 0 0 0 1 2 2 2
  spline S25 degree 2 poles (-10.9019, -3.6681) (-10.9019, -3.5044) (-10.957, -3.2937) (-11.0072, -3.2354) knots 0 0 0 1 2 2 2
  spline S26 degree 2 poles (-11.0072, -3.2354) (-11.0413, -3.1916) (-11.1288, -3.1543) (-11.179, -3.1543) knots 0 0 0 1 2 2 2
  spline S27 degree 2 poles (-11.179, -3.1543) (-11.2244, -3.1543) (-11.3087, -3.19) (-11.3476, -3.2354) knots 0 0 0 1 2 2 2
  spline S28 degree 2 poles (-11.3476, -3.2354) (-11.3816, -3.2743) (-11.4303, -3.425) (-11.4303, -3.5141) knots 0 0 0 1 2 2 2
  spline S29 degree 2 poles (-11.4303, -3.5141) (-11.4303, -3.6114) (-11.38, -3.7362) (-11.3379, -3.7735) knots 0 0 0 1 2 2 2
  spline S30 degree 2 poles (-11.3379, -3.7735) (-11.2941, -3.8107) (-11.1855, -3.8399) (-11.1175, -3.8399) knots 0 0 0 1 2 2 2
  spline S31 degree 2 poles (-11.1175, -3.8399) (-11.0607, -3.8399) (-10.9424, -3.8091) (-10.9051, -3.7929) knots 0 0 0 1 2 2 2
  spline S32 degree 2 poles (-10.9051, -3.7929) (-10.9051, -3.7783) (-10.9019, -3.7232) (-10.9019, -3.6681) knots 0 0 0 1 2 2 2
  line L10 (-8.6896, -4.8545) -> (-10.0105, -4.8545)
  line L11 (-10.0105, -4.8545) -> (-10.0105, -4.506)
  line L12 (-10.0105, -4.506) -> (-9.5891, -4.506)
  line L13 (-9.5891, -4.506) -> (-9.5891, -3.4477)
  line L14 (-9.5891, -3.4477) -> (-10.0105, -3.4477)
  line L15 (-10.0105, -3.4477) -> (-10.0105, -3.1219)
  spline S33 degree 2 poles (-10.0105, -3.1219) (-9.9181, -3.1219) (-9.735, -3.0976) (-9.6799, -3.0717) knots 0 0 0 1 2 2 2
  spline S34 degree 2 poles (-9.6799, -3.0717) (-9.6166, -3.0393) (-9.5453, -2.9307) (-9.5389, -2.8496) knots 0 0 0 1 2 2 2
  line L16 (-9.5389, -2.8496) -> (-9.1012, -2.8496)
  line L17 (-9.1012, -2.8496) -> (-9.1012, -4.506)
  line L18 (-9.1012, -4.506) -> (-8.6896, -4.506)
  line L19 (-8.6896, -4.506) -> (-8.6896, -4.8545)
  spline S35 degree 2 poles (-4.0769, -3.8545) (-4.0769, -4.3407) (-4.5956, -4.8966) (-5.0461, -4.8966) knots 0 0 0 1 2 2 2
  spline S36 degree 2 poles (-5.0461, -4.8966) (-5.4983, -4.8966) (-6.0137, -4.3342) (-6.0137, -3.8545) knots 0 0 0 1 2 2 2
  spline S37 degree 2 poles (-6.0137, -3.8545) (-6.0137, -3.3731) (-5.4983, -2.8124) (-5.0461, -2.8124) knots 0 0 0 1 2 2 2
  spline S38 degree 2 poles (-5.0461, -2.8124) (-4.5956, -2.8124) (-4.0769, -3.3699) (-4.0769, -3.8545) knots 0 0 0 1 2 2 2
  spline S39 degree 2 poles (-4.5956, -3.8545) (-4.5956, -3.6746) (-4.6685, -3.4234) (-4.7317, -3.344) knots 0 0 0 1 2 2 2
  spline S40 degree 2 poles (-4.7317, -3.344) (-4.7949, -3.2613) (-4.957, -3.19) (-5.0445, -3.19) knots 0 0 0 1 2 2 2
  spline S41 degree 2 poles (-5.0445, -3.19) (-5.1369, -3.19) (-5.2876, -3.2564) (-5.3573, -3.3407) knots 0 0 0 1 2 2 2
  spline S42 degree 2 poles (-5.3573, -3.3407) (-5.4189, -3.4185) (-5.4951, -3.6762) (-5.4951, -3.8545) knots 0 0 0 1 2 2 2
  spline S43 degree 2 poles (-5.4951, -3.8545) (-5.4951, -4.0393) (-5.4222, -4.2824) (-5.3589, -4.365) knots 0 0 0 1 2 2 2
  spline S44 degree 2 poles (-5.3589, -4.365) (-5.2957, -4.4477) (-5.132, -4.519) (-5.0445, -4.519) knots 0 0 0 1 2 2 2
  spline S45 degree 2 poles (-5.0445, -4.519) (-4.9554, -4.519) (-4.7901, -4.4428) (-4.7301, -4.3618) knots 0 0 0 1 2 2 2
  spline S46 degree 2 poles (-4.7301, -4.3618) (-4.6653, -4.2743) (-4.5956, -4.0425) (-4.5956, -3.8545) knots 0 0 0 1 2 2 2
  line L20 (-2.4448, -4.8545) -> (-3.7787, -4.8545)
  line L21 (-3.7787, -4.8545) -> (-3.7787, -2.8545)
  line L22 (-3.7787, -2.8545) -> (-3.2763, -2.8545)
  line L23 (-3.2763, -2.8545) -> (-3.2763, -4.4736)
  line L24 (-3.2763, -4.4736) -> (-2.4448, -4.4736)
  line L25 (-2.4448, -4.4736) -> (-2.4448, -4.8545)
  line L26 (-2.205, -4.8545) -> (-2.205, -2.8545)
  line L27 (-2.205, -2.8545) -> (-0.8533, -2.8545)
  line L28 (-0.8533, -2.8545) -> (-0.8533, -3.2354)
  line L29 (-0.8533, -3.2354) -> (-1.7058, -3.2354)
  line L30 (-1.7058, -3.2354) -> (-1.7058, -3.5871)
  line L31 (-1.7058, -3.5871) -> (-0.9197, -3.5871)
  line L32 (-0.9197, -3.5871) -> (-0.9197, -3.968)
  line L33 (-0.9197, -3.968) -> (-1.7058, -3.968)
  line L34 (-1.7058, -3.968) -> (-1.7058, -4.4736)
  line L35 (-1.7058, -4.4736) -> (-0.8533, -4.4736)
  line L36 (-0.8533, -4.4736) -> (-0.8533, -4.8545)
  line L37 (-0.8533, -4.8545) -> (-2.205, -4.8545)
  spline S47 degree 2 poles (1.2715, -3.8561) (1.2715, -4.1365) (1.0268, -4.5774) (0.8404, -4.6957) knots 0 0 0 1 2 2 2
  spline S48 degree 2 poles (0.8404, -4.6957) (0.6848, -4.7962) (0.3185, -4.8545) (0.1127, -4.8545) knots 0 0 0 1 2 2 2
  line L38 (0.1127, -4.8545) -> (-0.5129, -4.8545)
  line L39 (-0.5129, -4.8545) -> (-0.5129, -2.8545)
  line L40 (-0.5129, -2.8545) -> (0.1062, -2.8545)
  spline S49 degree 2 poles (0.1062, -2.8545) (0.3169, -2.8545) (0.6848, -2.908) (0.8469, -3.0117) knots 0 0 0 1 2 2 2
  spline S50 degree 2 poles (0.8469, -3.0117) (1.043, -3.1381) (1.2715, -3.566) (1.2715, -3.8561) knots 0 0 0 1 2 2 2
  spline S51 degree 2 poles (0.7561, -3.8529) (0.7561, -3.6552) (0.62, -3.3731) (0.4806, -3.2937) knots 0 0 0 1 2 2 2
  spline S52 degree 2 poles (0.4806, -3.2937) (0.3785, -3.2386) (0.1548, -3.2273) (-0.0008, -3.2273) knots 0 0 0 1 2 2 2
  line L41 (-0.0008, -3.2273) -> (-0.0105, -3.2273)
  line L42 (-0.0105, -3.2273) -> (-0.0105, -4.4801)
  line L43 (-0.0105, -4.4801) -> (-0.0008, -4.4801)
  spline S53 degree 2 poles (-0.0008, -4.4801) (0.1678, -4.4801) (0.3996, -4.4688) (0.5049, -4.4023) knots 0 0 0 1 2 2 2
  spline S54 degree 2 poles (0.5049, -4.4023) (0.6281, -4.3245) (0.7561, -4.0506) (0.7561, -3.8529) knots 0 0 0 1 2 2 2
  point P0 (0, 0)
  constraints: 2 other
extrude "Extrusion16" add sketch "Sketch16" along normal blind 0.1 separate body
sketch "Sketch17" plane through (0, 0, 0) normal (0, 0, -1) x (-1, 0, 0)
  line L0 (-4.2318, 4.4692) -> (-4.2318, 5.3849)
  line L1 (-4.2318, 5.3849) -> (-2.2161, 5.3849)
  line L2 (-2.2161, 5.3849) -> (-2.2161, 4.4692)
  line L3 (-3.3239, 4.4692) -> (-4.2318, 4.4692)
  line L4 (-2.2161, 4.4692) -> (-4.2318, 4.4692)
  line L5 (-4.2318, 4.4692) -> (-4.2318, 5.3849)
  line L6 (-14.2388, 5.3849) -> (-12.2231, 5.3849)
  line L7 (-12.2231, 5.3849) -> (-12.2231, 4.4692)
  line L8 (-12.2231, 4.4692) -> (-14.2388, 4.4692)
  line L9 (-14.2388, 4.4692) -> (-14.2388, 5.3849)
  line L10 (-14.2388, 1.8305) -> (-12.2231, 1.8305)
  line L11 (-12.2231, 1.8305) -> (-12.2231, 0.9148)
  line L12 (-12.2231, 0.9148) -> (-14.2388, 0.9148)
  line L13 (-14.2388, 0.9148) -> (-14.2388, 1.8305)
  line L14 (-12.2981, 5.3099) -> (-14.1638, 5.3099)
  line L15 (-14.1638, 5.3099) -> (-14.1638, 4.5442)
  line L16 (-14.1638, 4.5442) -> (-12.2981, 4.5442)
  line L17 (-12.2981, 4.5442) -> (-12.2981, 5.3099)
  line L18 (-12.2981, 1.7555) -> (-14.1638, 1.7555)
  line L19 (-14.1638, 1.7555) -> (-14.1638, 0.9898)
  line L20 (-14.1638, 0.9898) -> (-12.2981, 0.9898)
  line L21 (-12.2981, 0.9898) -> (-12.2981, 1.7555)
  point P0 (0, 0)
  dimension "d115" = 0.075
  dimension "d116" = 0.075
  constraints: 40 end point, 10 perpendicular, 3 horizontal, 1 collinear, 6 other
  measures "d115" distance between parallel lines of L6 L14
  measures "d116" distance between parallel lines of L10 L18
extrude "Extrusion17" add sketch "Sketch17" along normal up to surface (1 mm away) separate body contours L17 L16 L15 L14 | L21 L20 L19 L18
chamfer "Chamfer5" distance 0.1 angle 45 8 edges at (14.1638, 4.9271, -1) (13.2309, 5.3099, -1) (13.2309, 4.5442, -1) (12.2981, 4.9271, -1) (13.2309, 1.7555, -1) (14.1638, 1.3726, -1) (13.2309, 0.9898, -1) (12.2981, 1.3726, -1)
sketch "Sketch18" plane through (0, 0, 0) normal (0, 0, -1) x (-1, 0, 0)
  line L0 (-12.2518, 5.4667) -> (-10.648, 5.4667) construction
  line L1 (-10.648, 5.4667) -> (-10.648, 4.4456) construction
  line L2 (-10.648, 4.4456) -> (-12.2518, 4.4456) construction
  line L3 (-12.2518, 4.4456) -> (-12.2518, 5.4667) construction
  line L4 (-12.2148, 1.9063) -> (-10.4206, 1.9063) construction
  line L5 (-10.4206, 1.9063) -> (-10.4206, 0.8666) construction
  line L6 (-10.4206, 0.8666) -> (-12.2148, 0.8666) construction
  line L7 (-12.2148, 0.8666) -> (-12.2148, 1.9063) construction
  line L8 (-12.1655, 3.8775) -> (-10.2304, 3.8775) construction
  line L9 (-10.2304, 3.8775) -> (-10.2304, 2.5728) construction
  line L10 (-10.2304, 2.5728) -> (-12.1655, 2.5728) construction
  line L11 (-12.1655, 2.5728) -> (-12.1655, 3.8775) construction
  line L12 (-11.2242, 4.4667) -> (-11.5297, 4.4667)
  line L13 (-11.5297, 4.4667) -> (-11.8077, 4.8338)
  line L14 (-11.8077, 4.8338) -> (-11.8984, 4.8338)
  line L15 (-11.8984, 4.8338) -> (-11.8984, 4.4667)
  line L16 (-11.8984, 4.4667) -> (-12.148, 4.4667)
  line L17 (-12.148, 4.4667) -> (-12.148, 5.4667)
  line L18 (-12.148, 5.4667) -> (-11.7461, 5.4667)
  spline S0 degree 2 poles (-11.7461, 5.4667) (-11.6626, 5.4667) (-11.5394, 5.4456) (-11.4868, 5.4132) knots 0 0 0 1 2 2 2
  spline S1 degree 2 poles (-11.4868, 5.4132) (-11.4333, 5.3792) (-11.3701, 5.273) (-11.3701, 5.192) knots 0 0 0 1 2 2 2
  spline S2 degree 2 poles (-11.3701, 5.192) (-11.3701, 5.0777) (-11.4738, 4.9343) (-11.5605, 4.8921) knots 0 0 0 1 2 2 2
  line L19 (-11.5605, 4.8921) -> (-11.2242, 4.4667)
  spline S3 degree 2 poles (-11.6278, 5.1604) (-11.6278, 5.1985) (-11.657, 5.2528) (-11.6902, 5.2673) knots 0 0 0 1 2 2 2
  spline S4 degree 2 poles (-11.6902, 5.2673) (-11.7137, 5.2771) (-11.7712, 5.2827) (-11.8142, 5.2827) knots 0 0 0 1 2 2 2
  line L20 (-11.8142, 5.2827) -> (-11.8984, 5.2827)
  line L21 (-11.8984, 5.2827) -> (-11.8984, 5.0137)
  line L22 (-11.8984, 5.0137) -> (-11.8263, 5.0137)
  spline S5 degree 2 poles (-11.8263, 5.0137) (-11.7745, 5.0137) (-11.7007, 5.0267) (-11.6756, 5.0469) knots 0 0 0 1 2 2 2
  spline S6 degree 2 poles (-11.6756, 5.0469) (-11.6513, 5.0664) (-11.6278, 5.1182) (-11.6278, 5.1604) knots 0 0 0 1 2 2 2
  spline S7 degree 2 poles (-10.4398, 4.8054) (-10.4398, 4.7268) (-10.4933, 4.5939) (-10.5459, 4.5461) knots 0 0 0 1 2 2 2
  spline S8 degree 2 poles (-10.5459, 4.5461) (-10.5986, 4.4983) (-10.7429, 4.4456) (-10.8482, 4.4456) knots 0 0 0 1 2 2 2
  spline S9 degree 2 poles (-10.8482, 4.4456) (-10.96, 4.4464) (-11.1205, 4.4829) (-11.1732, 4.5064) knots 0 0 0 1 2 2 2
  line L23 (-11.1732, 4.5064) -> (-11.1732, 4.7244)
  line L24 (-11.1732, 4.7244) -> (-11.1505, 4.7244)
  spline S10 degree 2 poles (-11.1505, 4.7244) (-11.131, 4.7139) (-11.084, 4.6863) (-11.0459, 4.6717) knots 0 0 0 1 2 2 2
  spline S11 degree 2 poles (-11.0459, 4.6717) (-11.0103, 4.6579) (-10.9365, 4.6393) (-10.892, 4.6393) knots 0 0 0 1 2 2 2
  spline S12 degree 2 poles (-10.892, 4.6393) (-10.8531, 4.6393) (-10.7623, 4.6587) (-10.7347, 4.6847) knots 0 0 0 1 2 2 2
  spline S13 degree 2 poles (-10.7347, 4.6847) (-10.7145, 4.7049) (-10.6918, 4.7544) (-10.6918, 4.7957) knots 0 0 0 1 2 2 2
  spline S14 degree 2 poles (-10.6918, 4.7957) (-10.6918, 4.8314) (-10.721, 4.8816) (-10.7445, 4.897) knots 0 0 0 1 2 2 2
  spline S15 degree 2 poles (-10.7445, 4.897) (-10.7785, 4.9197) (-10.8758, 4.9327) (-10.9106, 4.9327) knots 0 0 0 1 2 2 2
  spline S16 degree 2 poles (-10.9106, 4.9327) (-10.9657, 4.9327) (-11.0702, 4.9148) (-11.1083, 4.9051) knots 0 0 0 1 2 2 2
  line L25 (-11.1083, 4.9051) -> (-11.1302, 4.9051)
  line L26 (-11.1302, 4.9051) -> (-11.1302, 5.4667)
  line L27 (-11.1302, 5.4667) -> (-10.4673, 5.4667)
  line L28 (-10.4673, 5.4667) -> (-10.4673, 5.2779)
  line L29 (-10.4673, 5.2779) -> (-10.8928, 5.2779)
  line L30 (-10.8928, 5.2779) -> (-10.8928, 5.1117)
  spline S17 degree 2 poles (-10.8928, 5.1117) (-10.8725, 5.1134) (-10.8166, 5.115) (-10.8012, 5.115) knots 0 0 0 1 2 2 2
  spline S18 degree 2 poles (-10.8012, 5.115) (-10.7291, 5.115) (-10.6075, 5.0858) (-10.5597, 5.0558) knots 0 0 0 1 2 2 2
  spline S19 degree 2 poles (-10.5597, 5.0558) (-10.503, 5.0186) (-10.4398, 4.8946) (-10.4398, 4.8054) knots 0 0 0 1 2 2 2
  spline S20 degree 2 poles (-11.1534, 2.5922) (-11.1939, 2.5825) (-11.2749, 2.5728) (-11.3616, 2.5728) knots 0 0 0 1 2 2 2
  spline S21 degree 2 poles (-11.3616, 2.5728) (-11.4402, 2.5728) (-11.5513, 2.6125) (-11.5885, 2.6489) knots 0 0 0 1 2 2 2
  spline S22 degree 2 poles (-11.5885, 2.6489) (-11.625, 2.6846) (-11.6623, 2.7818) (-11.6647, 2.8386) knots 0 0 0 1 2 2 2
  spline S23 degree 2 poles (-11.6647, 2.8386) (-11.8762, 2.8483) (-12.1201, 3.123) (-12.1201, 3.3564) knots 0 0 0 1 2 2 2
  spline S24 degree 2 poles (-12.1201, 3.3564) (-12.1201, 3.5971) (-11.8624, 3.8775) (-11.6364, 3.8775) knots 0 0 0 1 2 2 2
  spline S25 degree 2 poles (-11.6364, 3.8775) (-11.4111, 3.8775) (-11.1518, 3.5987) (-11.1518, 3.3564) knots 0 0 0 1 2 2 2
  spline S26 degree 2 poles (-11.1518, 3.3564) (-11.1518, 3.1797) (-11.2984, 2.9269) (-11.433, 2.8734) knots 0 0 0 1 2 2 2
  spline S27 degree 2 poles (-11.433, 2.8734) (-11.4313, 2.7997) (-11.3689, 2.7438) (-11.2911, 2.7438) knots 0 0 0 1 2 2 2
  spline S28 degree 2 poles (-11.2911, 2.7438) (-11.2603, 2.7438) (-11.1931, 2.7616) (-11.1785, 2.7697) knots 0 0 0 1 2 2 2
  line L31 (-11.1785, 2.7697) -> (-11.1534, 2.7697)
  line L32 (-11.1534, 2.7697) -> (-11.1534, 2.5922)
  spline S29 degree 2 poles (-11.4783, 3.1036) (-11.4459, 3.1473) (-11.4111, 3.2632) (-11.4111, 3.3572) knots 0 0 0 1 2 2 2
  spline S30 degree 2 poles (-11.4111, 3.3572) (-11.4111, 3.4463) (-11.4475, 3.572) (-11.4791, 3.6125) knots 0 0 0 1 2 2 2
  spline S31 degree 2 poles (-11.4791, 3.6125) (-11.5107, 3.653) (-11.5918, 3.6886) (-11.6355, 3.6886) knots 0 0 0 1 2 2 2
  spline S32 degree 2 poles (-11.6355, 3.6886) (-11.6817, 3.6886) (-11.7571, 3.6554) (-11.7919, 3.6133) knots 0 0 0 1 2 2 2
  spline S33 degree 2 poles (-11.7919, 3.6133) (-11.8227, 3.5744) (-11.8608, 3.4455) (-11.8608, 3.3564) knots 0 0 0 1 2 2 2
  spline S34 degree 2 poles (-11.8608, 3.3564) (-11.8608, 3.2648) (-11.8244, 3.1433) (-11.7928, 3.1019) knots 0 0 0 1 2 2 2
  spline S35 degree 2 poles (-11.7928, 3.1019) (-11.7612, 3.0606) (-11.6793, 3.025) (-11.6355, 3.025) knots 0 0 0 1 2 2 2
  spline S36 degree 2 poles (-11.6355, 3.025) (-11.591, 3.025) (-11.5083, 3.063) (-11.4783, 3.1036) knots 0 0 0 1 2 2 2
  line L33 (-10.3146, 2.8564) -> (-10.9751, 2.8564)
  line L34 (-10.9751, 2.8564) -> (-10.9751, 3.0306)
  line L35 (-10.9751, 3.0306) -> (-10.7644, 3.0306)
  line L36 (-10.7644, 3.0306) -> (-10.7644, 3.5598)
  line L37 (-10.7644, 3.5598) -> (-10.9751, 3.5598)
  line L38 (-10.9751, 3.5598) -> (-10.9751, 3.7227)
  spline S37 degree 2 poles (-10.9751, 3.7227) (-10.9289, 3.7227) (-10.8373, 3.7348) (-10.8098, 3.7478) knots 0 0 0 1 2 2 2
  spline S38 degree 2 poles (-10.8098, 3.7478) (-10.7782, 3.764) (-10.7425, 3.8183) (-10.7393, 3.8588) knots 0 0 0 1 2 2 2
  line L39 (-10.7393, 3.8588) -> (-10.5205, 3.8588)
  line L40 (-10.5205, 3.8588) -> (-10.5205, 3.0306)
  line L41 (-10.5205, 3.0306) -> (-10.3146, 3.0306)
  line L42 (-10.3146, 3.0306) -> (-10.3146, 2.8564)
  spline S39 degree 2 poles (-11.68, 0.8666) (-11.9052, 0.8666) (-12.1694, 1.1389) (-12.1694, 1.3853) knots 0 0 0 1 2 2 2
  spline S40 degree 2 poles (-12.1694, 1.3853) (-12.1694, 1.6227) (-11.9044, 1.9055) (-11.6792, 1.9055) knots 0 0 0 1 2 2 2
  spline S41 degree 2 poles (-11.6792, 1.9055) (-11.62, 1.9055) (-11.5244, 1.8917) (-11.4806, 1.8804) knots 0 0 0 1 2 2 2
  spline S42 degree 2 poles (-11.4806, 1.8804) (-11.4466, 1.8699) (-11.3663, 1.835) (-11.3412, 1.8221) knots 0 0 0 1 2 2 2
  line L43 (-11.3412, 1.8221) -> (-11.3412, 1.5838)
  line L44 (-11.3412, 1.5838) -> (-11.3663, 1.5838)
  spline S43 degree 2 poles (-11.3663, 1.5838) (-11.385, 1.6) (-11.4401, 1.6454) (-11.4749, 1.6665) knots 0 0 0 1 2 2 2
  spline S44 degree 2 poles (-11.4749, 1.6665) (-11.5098, 1.6883) (-11.5933, 1.7183) (-11.6394, 1.7183) knots 0 0 0 1 2 2 2
  spline S45 degree 2 poles (-11.6394, 1.7183) (-11.6937, 1.7183) (-11.7837, 1.6843) (-11.825, 1.6413) knots 0 0 0 1 2 2 2
  spline S46 degree 2 poles (-11.825, 1.6413) (-11.8623, 1.6033) (-11.9101, 1.4728) (-11.9101, 1.3845) knots 0 0 0 1 2 2 2
  spline S47 degree 2 poles (-11.9101, 1.3845) (-11.9101, 1.2913) (-11.8607, 1.164) (-11.8202, 1.1251) knots 0 0 0 1 2 2 2
  spline S48 degree 2 poles (-11.8202, 1.1251) (-11.7813, 1.087) (-11.6856, 1.0538) (-11.6378, 1.0538) knots 0 0 0 1 2 2 2
  spline S49 degree 2 poles (-11.6378, 1.0538) (-11.5884, 1.0538) (-11.4984, 1.087) (-11.4676, 1.1073) knots 0 0 0 1 2 2 2
  spline S50 degree 2 poles (-11.4676, 1.1073) (-11.4336, 1.1276) (-11.3826, 1.1705) (-11.3639, 1.1875) knots 0 0 0 1 2 2 2
  line L45 (-11.3639, 1.1875) -> (-11.3412, 1.1875)
  line L46 (-11.3412, 1.1875) -> (-11.3412, 0.9525)
  spline S51 degree 2 poles (-11.3412, 0.9525) (-11.3688, 0.9396) (-11.4409, 0.9071) (-11.4798, 0.8958) knots 0 0 0 1 2 2 2
  spline S52 degree 2 poles (-11.4798, 0.8958) (-11.5268, 0.8812) (-11.6086, 0.8666) (-11.68, 0.8666) knots 0 0 0 1 2 2 2
  spline S53 degree 2 poles (-10.4863, 1.442) (-10.4863, 1.3148) (-10.5454, 1.1024) (-10.6078, 1.0263) knots 0 0 0 1 2 2 2
  spline S54 degree 2 poles (-10.6078, 1.0263) (-10.6727, 0.9493) (-10.8639, 0.8666) (-11.0033, 0.8666) knots 0 0 0 1 2 2 2
  spline S55 degree 2 poles (-11.0033, 0.8666) (-11.0503, 0.8666) (-11.1524, 0.8788) (-11.1694, 0.8836) knots 0 0 0 1 2 2 2
  line L47 (-11.1694, 0.8836) -> (-11.1694, 1.0798)
  line L48 (-11.1694, 1.0798) -> (-11.15, 1.0798)
  spline S56 degree 2 poles (-11.15, 1.0798) (-11.1313, 1.07) (-11.0616, 1.049) (-11.0009, 1.049) knots 0 0 0 1 2 2 2
  spline S57 degree 2 poles (-11.0009, 1.049) (-10.9514, 1.049) (-10.8599, 1.0749) (-10.8274, 1.1033) knots 0 0 0 1 2 2 2
  spline S58 degree 2 poles (-10.8274, 1.1033) (-10.7926, 1.1332) (-10.7472, 1.2216) (-10.7391, 1.288) knots 0 0 0 1 2 2 2
  spline S59 degree 2 poles (-10.7391, 1.288) (-10.7926, 1.2548) (-10.885, 1.2191) (-10.9539, 1.2191) knots 0 0 0 1 2 2 2
  spline S60 degree 2 poles (-10.9539, 1.2191) (-11.0049, 1.2191) (-11.0997, 1.2467) (-11.1386, 1.2759) knots 0 0 0 1 2 2 2
  spline S61 degree 2 poles (-11.1386, 1.2759) (-11.1905, 1.3156) (-11.2513, 1.4428) (-11.2513, 1.5433) knots 0 0 0 1 2 2 2
  spline S62 degree 2 poles (-11.2513, 1.5433) (-11.2513, 1.6219) (-11.1978, 1.754) (-11.1492, 1.8026) knots 0 0 0 1 2 2 2
  spline S63 degree 2 poles (-11.1492, 1.8026) (-11.1005, 1.8512) (-10.9595, 1.9063) (-10.8728, 1.9063) knots 0 0 0 1 2 2 2
  spline S64 degree 2 poles (-10.8728, 1.9063) (-10.7853, 1.9063) (-10.65, 1.8577) (-10.6014, 1.8067) knots 0 0 0 1 2 2 2
  spline S65 degree 2 poles (-10.6014, 1.8067) (-10.5446, 1.7499) (-10.4863, 1.57) (-10.4863, 1.442) knots 0 0 0 1 2 2 2
  spline S66 degree 2 poles (-10.7351, 1.4793) (-10.7351, 1.5611) (-10.7626, 1.6665) (-10.7877, 1.6956) knots 0 0 0 1 2 2 2
  spline S67 degree 2 poles (-10.7877, 1.6956) (-10.8048, 1.7175) (-10.8485, 1.7362) (-10.8736, 1.7362) knots 0 0 0 1 2 2 2
  spline S68 degree 2 poles (-10.8736, 1.7362) (-10.8963, 1.7362) (-10.9385, 1.7183) (-10.9579, 1.6956) knots 0 0 0 1 2 2 2
  spline S69 degree 2 poles (-10.9579, 1.6956) (-10.9749, 1.6762) (-10.9992, 1.6008) (-10.9992, 1.5563) knots 0 0 0 1 2 2 2
  spline S70 degree 2 poles (-10.9992, 1.5563) (-10.9992, 1.5076) (-10.9741, 1.4452) (-10.9531, 1.4266) knots 0 0 0 1 2 2 2
  spline S71 degree 2 poles (-10.9531, 1.4266) (-10.9312, 1.408) (-10.8769, 1.3934) (-10.8428, 1.3934) knots 0 0 0 1 2 2 2
  spline S72 degree 2 poles (-10.8428, 1.3934) (-10.8145, 1.3934) (-10.7553, 1.4088) (-10.7367, 1.4169) knots 0 0 0 1 2 2 2
  spline S73 degree 2 poles (-10.7367, 1.4169) (-10.7367, 1.4242) (-10.7351, 1.4517) (-10.7351, 1.4793) knots 0 0 0 1 2 2 2
  point P0 (0, 0)
  constraints: 6 other
extrude "Extrusion18" add sketch "Sketch18" along normal blind 0.1 separate body
sketch "Sketch19" plane through (0, 0, 0) normal (0, 0, -1) x (-1, 0, 0)
  line L0 (-14.7777, 2.1542) -> (-14.7777, 4.2325)
  line L1 (-14.7777, 4.2325) -> (-13.5496, 4.2325)
  line L2 (-13.5496, 4.2325) -> (-13.5496, 2.1542)
  line L3 (-13.5496, 2.1542) -> (-14.7777, 2.1542)
  line L4 (-14.7777, 2.1542) -> (-13.5496, 4.2325) construction
  line L5 (-14.7777, 4.2325) -> (-13.5496, 2.1542) construction
  point P0 (0, 0)
  point P1 (-14.1636, 3.1933)
  constraints: 12 end point, 2 midpoint, 2 parallel, 1 perpendicular, 1 vertical
extrude "Extrusion19" add sketch "Sketch19" along normal up to surface (1 mm away) separate body
chamfer "Chamfer6" distance 0.1 angle 45 4 edges at (14.7777, 3.1933, -1) (13.5496, 3.1933, -1) (14.1636, 4.2325, -1) (14.1636, 2.1542, -1)